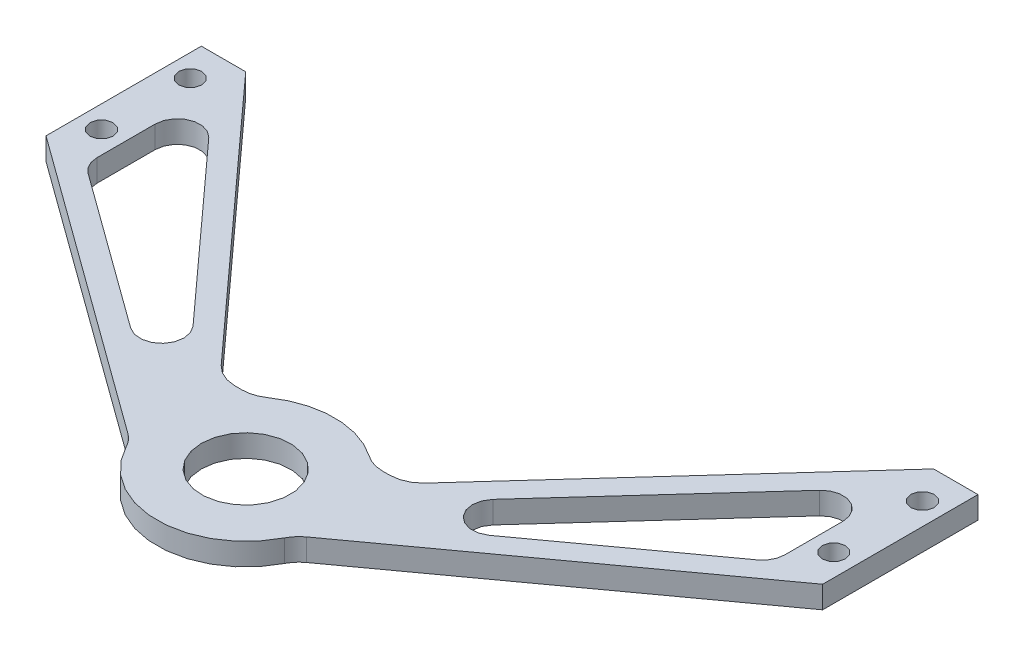
# Autodesk Inventor part: shoulder
Saved by Autodesk Inventor 2018 (Build 220112000, 112)
## iProperties
Created: 2018-09-03
Part Number: shoulder
Material: 一般
Document SubType Name: Modeling
Designer: y6tada
Density: 1 g/cm^3
Appearance: 既定
Author: y6tada
Autodesk Inventor part; units mm, degrees
ref_plane "YZ Plane" through (0, 0, 0) normal (1, 0, 0) x (0, 1, 0)
ref_plane "XZ Plane" through (0, 0, 0) normal (0, 1, 0) x (-1, 0, 0)
ref_plane "XY Plane" through (0, 0, 0) normal (0, 0, 1) x (1, 0, 0)
sketch "スケッチ1" plane through (0, 0, 0) normal (0, 1, 0) x (-1, 0, 0)
  arc A0 (0, -8) -> (4.5997, -6.5455) centre (0, 0) ccw
  line L0 (33, -28) -> (33, -20) construction
  line L1 (0, 0) -> (0, -13.0211) construction
  circle A1 centre (33, -28) radius 1.05
  circle A2 centre (33, -20) radius 1.05
  line L2 (31, -31) -> (9.1961, -6.9835)
  line L3 (31, -31) -> (35, -31)
  line L4 (35, -31) -> (35, -17)
  line L5 (35, -17) -> (8.0357, 2.5722)
  line L6 (31, -22.8462) -> (31, -17.5875)
  line L7 (30.1748, -15.969) -> (16.1748, -5.807)
  line L8 (13.5192, -8.7699) -> (27.5192, -24.1906)
  arc A3 (27.5192, -24.1906) -> (31, -22.8462) centre (29, -22.8462) ccw
  arc A4 (31, -17.5875) -> (30.1748, -15.969) centre (29, -17.5875) ccw
  arc A5 (16.1748, -5.807) -> (13.5192, -8.7699) centre (15, -7.4256) ccw
  line L9 (6.9749, -6) -> (6.3246, -6)
  arc A6 (7.1258, 3.6364) -> (0, 8) centre (0, 0) ccw
  line L10 (0, 8) -> (0, 0) construction
  arc A7 (6.3246, -6) -> (4.5997, -6.5455) centre (6.3246, -9) ccw
  arc A8 (7.1258, 3.6364) -> (8.0357, 2.5722) centre (9.798, 5) ccw
  arc A9 (9.1961, -6.9835) -> (6.9749, -6) centre (6.9749, -9) ccw
  arc A10 (-4.5997, -6.5455) -> (0, -8) centre (0, 0) ccw
  line L11 (-33, -28) -> (-33, -20) construction
  circle A11 centre (-33, -28) radius 1.05
  circle A12 centre (-33, -20) radius 1.05
  line L12 (-31, -31) -> (-9.1961, -6.9835)
  line L13 (-31, -31) -> (-35, -31)
  line L14 (-35, -31) -> (-35, -17)
  line L15 (-35, -17) -> (-8.0357, 2.5722)
  line L16 (-31, -22.8462) -> (-31, -17.5875)
  line L17 (-30.1748, -15.969) -> (-16.1748, -5.807)
  line L18 (-13.5192, -8.7699) -> (-27.5192, -24.1906)
  arc A13 (-31, -22.8462) -> (-27.5192, -24.1906) centre (-29, -22.8462) ccw
  arc A14 (-30.1748, -15.969) -> (-31, -17.5875) centre (-29, -17.5875) ccw
  arc A15 (-13.5192, -8.7699) -> (-16.1748, -5.807) centre (-15, -7.4256) ccw
  line L19 (-6.9749, -6) -> (-6.3246, -6)
  arc A16 (0, 8) -> (-7.1258, 3.6364) centre (0, 0) ccw
  arc A17 (-4.5997, -6.5455) -> (-6.3246, -6) centre (-6.3246, -9) ccw
  arc A18 (-8.0357, 2.5722) -> (-7.1258, 3.6364) centre (-9.798, 5) ccw
  arc A19 (-6.9749, -6) -> (-9.1961, -6.9835) centre (-6.9749, -9) ccw
  circle A20 centre (0, 0) radius 4
  point P0 (5.2915, -6)
  point P1 (-5.2915, -6)
  dimension "d0" = 2.1
  dimension "d1" = 8
  dimension "d2" = 4
  dimension "d3" = 3
  dimension "d4" = 3
  dimension "d5" = 70
  dimension "d6" = 2
  dimension "d7" = 2
  dimension "d8" = 2
  dimension "d10" = 8
  dimension "d11" = 3
  dimension "d12" = 20
  dimension "d13" = 6
  dimension "d14" = 5
  dimension "d15" = 15
  dimension "d16" = 8
  constraints: 40 end point, 34 point on circle, 26 symmetric about line, 21 centre point, 12 tangent, 6 coincident, 6 equal radius, 5 point on line, 3 vertical, 2 horizontal, 2 parallel, 1 collinear, 1 concentric, 1 perpendicular, 11 other
  measures "d0" diameter of A1
  measures "d1" distance of L0.start L0.end
  measures "d2" distance between parallel lines of L4 L6
  measures "d3" distance from line of L3 L0.start
  measures "d4" vertical distance of L4.end L0.end
  measures "d5" diameter of L4 L1
  measures "d6" distance between parallel lines of L2 L8
  measures "d7" distance between parallel lines of L5 L7
  measures "d8" radius of A3
  measures "d10" radius of A0
  measures "d11" radius of A7
  measures "d12" vertical distance of point (0, 0) L0.end
  measures "d13" distance from line of point (0, 0) L9
  measures "d14" vertical distance of point (0, 0) A8.centre
  measures "d15" distance from line of L10 A5.centre
  measures "d16" diameter of A20
extrude "押し出し1" add sketch "スケッチ1" along normal blind 2
